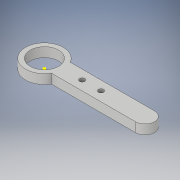
# Autodesk Inventor part: Part2
Saved by Autodesk Inventor 2019 (Build 230136000, 136)
## iProperties
Created: 2020-01-23
Part Number: Part2
Material: Generic
Document SubType Name: Modeling
Designer: pengj5
Density: 1 g/cm^3
Appearance: Default
Author: pengj5
Autodesk Inventor part; units mm, degrees
ref_plane "YZ Plane" through (0, 0, 0) normal (1, 0, 0) x (0, 1, 0)
ref_plane "XZ Plane" through (0, 0, 0) normal (0, 1, 0) x (-1, 0, 0)
ref_plane "XY Plane" through (0, 0, 0) normal (0, 0, 1) x (1, 0, 0)
sketch "Sketch1" plane through (0, 0, 0) normal (0, 1, 0) x (-1, 0, 0)
  point P0 (0, 0)
sketch "Sketch2" plane through (0, 0, 0) normal (0, 1, 0) x (-1, 0, 0)
  arc A0 (-25.9808, -15) -> (-25.9808, 15) centre (0, 0) ccw
  line L0 (-160, 15) -> (-25.9808, 15)
  arc A1 (-160, 15) -> (-160, -15) centre (-160, 0) ccw
  line L1 (-25.9808, -15) -> (-160, -15)
  dimension "d1" = 60
  dimension "d4" = 30
  constraints: 4 end point, 4 point on circle, 2 centre point
  measures "d1" diameter of A0
  measures "d4" distance of L1.end L0.start
extrude "Extrusion1" add sketch "Sketch2" along normal blind 15
sketch "Sketch3" plane through (0, 0, 0) normal (0, -1, 0) x (1, 0, 0)
  circle A0 centre (0, 0) radius 22.5
  circle A1 centre (60, 0) radius 4
  circle A2 centre (90, 0) radius 4
  dimension "d7" = 45
  dimension "d16" = 8
  dimension "d17" = 8
  constraints: 3 centre point, 1 coincident
  measures "d7" diameter of A0
  measures "d16" diameter of A1
  measures "d17" diameter of A2
extrude "Extrusion2" cut sketch "Sketch3" against normal blind 15
body "Solid1"
